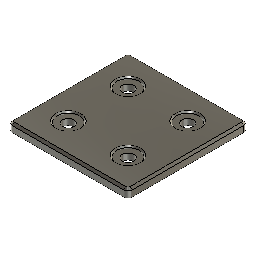
EXTRUSIONconnector (Autodesk Fusion 360 design; units mm, degrees)
Autodesk Fusion 360 part; units mm, degrees
sketch "Sketch1" plane through (0, 0, 0) normal (0, 0, 1) x (1, 0, 0)
  line L0 (30, 30) -> (-30, 30)
  line L1 (-30, 30) -> (-30, -30)
  line L2 (-30, -30) -> (30, -30)
  line L3 (30, -30) -> (30, 30)
  line L4 (30, 30) -> (-30, -30) construction
  line L5 (-30, 30) -> (30, -30) construction
  line L6 (-30, -30) -> (-15, -30) construction
  line L7 (-15, -30) -> (-15, -15) construction
  line L8 (-15, -15) -> (-30, -15) construction
  line L9 (-30, -15) -> (-30, -30) construction
  line L10 (-11, -3) -> (-19, -3)
  line L11 (-19, -3) -> (-19, -27)
  line L12 (-19, -27) -> (-11, -27)
  line L13 (-11, -27) -> (-11, -3)
  line L14 (-11, -3) -> (-19, -27) construction
  line L15 (-19, -3) -> (-11, -27) construction
  line L16 (-11, -7) -> (-19, -7)
  line L17 (-19, -7) -> (-19, -23)
  line L18 (-19, -23) -> (-11, -23)
  line L19 (-11, -23) -> (-11, -7)
  line L20 (-11, -7) -> (-19, -23) construction
  line L21 (-19, -7) -> (-11, -23) construction
  point P0 (-15, -15)
  point P1 (-15, -15)
  point P2 (-15, -15)
  dimension "d1" = 60
  dimension "d2" = 60
  dimension "d25" = 15
  dimension "d26" = 15
  dimension "d38" = 8
  dimension "d39" = 24
  dimension "d40" = 8
  dimension "d41" = 16
  constraint horizontal L0
  constraint perpendicular L0 L1
  constraint parallel L0 L2
  constraint parallel L1 L3
  constraint coincident L4 origin
  constraint coincident L5 origin
  constraint horizontal L6
  constraint vertical L7
  constraint horizontal L8
  constraint vertical L9
  constraint coincident P2 P1
  constraint horizontal L10
  constraint perpendicular L10 L11
  constraint parallel L10 L12
  constraint parallel L11 L13
  constraint coincident L14 P2
  constraint coincident L15 P2
  constraint horizontal L16
  constraint perpendicular L16 L17
  constraint parallel L16 L18
  constraint parallel L17 L19
  constraint coincident L20 P2
  constraint coincident L21 P2
  measures "d1" distance of L1.end L2.end
  measures "d2" distance of L0.end L1.end
  measures "d25" distance of L1.end L6.end
  measures "d26" distance of L1.end L8.end
  measures "d38" distance of L11.end L12.end
  measures "d39" distance of L10.end L11.end
  measures "d40" distance of L17.end L18.end
  measures "d41" distance of L16.end L17.end
extrude "Extrude1" add sketch "Sketch1" against normal blind 4 contours L0 L1 L2 L3 | L10 L11 L13 L16 | L11 L13 L16 L17 L18 L19 | L11 L12 L13 L18 in component "body"
hole "Hole2" at (-15, -15, 0) direction (0, 0, -1) diameter 6 depth 4 tip angle 118 counterbore diameter 11.5 counterbore depth 1 in component "body"
extrude "Extrude2" add sketch "Sketch1" against normal blind 2 from surface at -4 contours L10 L11 L13 L16 | L11 L12 L13 L18 in component "body"
chamfer "Chamfer4" distance 0.5 angle 45 2 faces at (-16.3333, -25.6667, -6) (-16.3333, -4.3333, -6) in component "body"
chamfer "Chamfer4" distance 0.6 angle 45 1 edges at (-20.3609, -12.9207, 0) in component "body"
pattern_linear "R-Pattern2" count 2 spacing 30 along (0, 1, 0) count 2 spacing 30 along (1, 0, 0) of "Hole2", "Extrude2", "Chamfer4" in component "body"
fillet "Fillet1" radius 2 4 edges at (-30, -30, -2) (30, -30, -2) (30, 30, -2) (-30, 30, -2) in component "body"
chamfer "Chamfer1" distance 1 distance2 1 8 edges at (0, -30, 0) (29.4142, -29.4142, 0) (30, 0, 0) (29.4142, 29.4142, 0) (0, 30, 0) (-29.4142, 29.4142, 0) (-30, 0, 0) (-29.4142, -29.4142, 0) measured on face at (-3.5603, 3.4484, 0) measured on face at (28.0952, -29.9977, -1.3333) measured on face at (-3.5603, 3.4484, 0) measured on face at (28.0952, 29.9977, -1.3333) measured on face at (-3.5603, 3.4484, 0) measured on face at (-29.9977, 28.0952, -1.3333) measured on face at (-3.5603, 3.4484, 0) measured on face at (-29.9977, -28.0952, -1.3333) in component "body"
component "body" placed x (1, 0, 0) y (0, 1, 0) z (0, 0, 1) at (0, 0, 0)
equation "d2 = unitY * size"
equation "size = 30 mm"
equation "unitX = 2"
equation "unitY = 2"
equation "d21 = unitY"
equation "d22 = unitX"
equation "d23 = size"
equation "d24 = -size"
equation "d25 = size / 2"
equation "d26 = size / 2"
